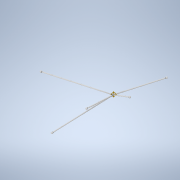
# Autodesk Inventor part: Coupler
Saved by Autodesk Inventor 2020.1 (Build 241239000, 239)
## iProperties
Created: 2019-10-25
Part Number: Coupler
Material: Generic
Document SubType Name: Modeling
Designer: sshel
Density: 1 g/cm^3
Appearance: Default
Mass: 190025 g
Surface Area: 74701 cm^2
Volume: 190025 cm^3
Author: sshel
Autodesk Inventor part; units mm, degrees
ref_plane "YZ Plane" through (0, 0, 0) normal (1, 0, 0) x (0, 1, 0)
ref_plane "XZ Plane" through (0, 0, 0) normal (0, 1, 0) x (-1, 0, 0)
ref_plane "XY Plane" through (0, 0, 0) normal (0, 0, 1) x (1, 0, 0)
ref_plane "Dyad1 plane" through (-2903, -72.8, 218.4) normal (-0.9968703, -0.024999, 0.0749971) x (0.0250696, -0.9996857, 0)
sketch "Sketch3" plane through (-2903, -72.8, 218.4) normal (-0.9968703, -0.024999, 0.0749971) x (0.0250696, -0.9996857, 0)
  circle A0 centre (0, 0) radius 50
  point P0 (0, 0)
  dimension "d16" = 50
  constraints: 1 centre point, 1 coincident
  measures "d16" radius of A0
sketch3d "import_point_3Dsketch"
  line L0 (-2903, -72.8, 218.4) -> (0, 0, 0)
sweep "Dyad1 rod" add profiles "Sketch3" path "import_point_3Dsketch"
sketch "Sketch2" plane through (-2903, -72.8, 218.4) normal (-0.9968703, -0.024999, 0.0749971) x (0.0250696, -0.9996857, 0)
  circle A0 centre (0, 0) radius 100
  line L0 (100, 0) -> (-100, 0)
  point P0 (0, 0)
  dimension "d17" = 100
  constraints: 2 end point, 2 point on circle, 1 centre point, 1 coincident, 1 horizontal, 1 midpoint
  measures "d17" radius of A0
revolve "Dyad1 joint" add sketch "Sketch2" angle 360 about axis through (-2900.493, -172.7686, 218.4) along (-0.0250696, 0.9996857, 0) separate body picked at (-20.1483, -40.7644) contours A0 L0
ref_plane "Dyad2 plane" through (-331.6, -2095.8, 1005.2) normal (-0.1412309, -0.892617, 0.4281223) x (0.9877132, -0.1562772, 0)
sketch "Sketch4" plane through (-331.6, -2095.8, 1005.2) normal (-0.1412309, -0.892617, 0.4281223) x (0.9877132, -0.1562772, 0)
  circle A0 centre (0, 0) radius 50
  dimension "d14" = 50
  constraints: 1 centre point, 1 coincident
  measures "d14" radius of A0
sketch3d "import_point_3Dsketch for Dyad2 rod"
  line L0 (-331.6, -2095.8, 1005.2) -> (0, 0, 0)
sweep "Dyad2 rod" add profiles "Sketch4" path "import_point_3Dsketch for Dyad2 rod" separate body
sketch "Sketch5" plane through (-331.6, -2095.8, 1005.2) normal (-0.1412309, -0.892617, 0.4281223) x (0.9877132, -0.1562772, 0)
  circle A0 centre (0, 0) radius 100
  line L0 (100, 0) -> (-100, 0)
  dimension "d11" = 100
  constraints: 2 end point, 2 point on circle, 1 centre point, 1 coincident, 1 horizontal, 1 midpoint
  measures "d11" radius of A0
revolve "Dyad2 joint" add sketch "Sketch5" angle 360 about axis through (-232.8287, -2111.4277, 1005.2) along (-0.9877132, 0.1562772, 0) picked at (-20.1483, -40.7644) bodies 2 contours A0 L0
ref_plane "Dyad3 plane" through (-5519.4, 1007.5, -1258) normal (-0.9599117, 0.1752203, -0.2187863) x (-0.1795708, -0.9837451, 0)
sketch "Sketch6" plane through (-5519.4, 1007.5, -1258) normal (-0.9599117, 0.1752203, -0.2187863) x (-0.1795708, -0.9837451, 0)
  circle A0 centre (0, 0) radius 50
  point P0 (0, 0)
  dimension "d18" = 50
  constraints: 1 centre point, 1 coincident
  measures "d18" radius of A0
sketch3d "import_point_3Dsketch for Dyad3 rod"
  line L0 (-5519.4, 1007.5, -1258) -> (0, 0, 0)
sweep "Dyad3 rod" add profiles "Sketch6" path "import_point_3Dsketch for Dyad3 rod" separate body
sketch "Sketch7" plane through (-5519.4, 1007.5, -1258) normal (-0.9599117, 0.1752203, -0.2187863) x (-0.1795708, -0.9837451, 0)
  circle A0 centre (0, 0) radius 100
  line L0 (100, 0) -> (-100, 0)
  point P0 (0, 0)
  dimension "d21" = 100
  constraints: 2 end point, 2 point on circle, 1 centre point, 1 coincident, 1 horizontal, 1 midpoint
  measures "d21" radius of A0
revolve "Dyad3 joint" add sketch "Sketch7" angle 360 about axis through (-5537.3571, 909.1255, -1258) along (0.1795708, 0.9837451, 0) picked at (-20.1483, -40.7644) bodies 2 contours A0 L0
ref_plane "Dyad4 plane" through (4188.4, -1511.9, 245.4) normal (0.9391702, -0.3390153, 0.0550264) x (0.3395297, 0.9405953, 0)
sketch "Sketch8" plane through (4188.4, -1511.9, 245.4) normal (0.9391702, -0.3390153, 0.0550264) x (0.3395297, 0.9405953, 0)
  circle A0 centre (0, 0) radius 50
  point P0 (0, 0)
  dimension "d23" = 50
  constraints: 1 centre point, 1 coincident
  measures "d23" radius of A0
sketch3d "import_point_3Dsketch for Dyad4 rod"
  line L0 (4188.4, -1511.9, 245.4) -> (0, 0, 0)
sweep "Dyad4 rod" add profiles "Sketch8" path "import_point_3Dsketch for Dyad4 rod" separate body
sketch "Sketch9" plane through (4188.4, -1511.9, 245.4) normal (0.9391702, -0.3390153, 0.0550264) x (0.3395297, 0.9405953, 0)
  circle A0 centre (0, 0) radius 100
  line L0 (100, 0) -> (-100, 0)
  point P0 (0, 0)
  dimension "d26" = 100
  constraints: 2 end point, 2 point on circle, 1 centre point, 1 coincident, 1 horizontal, 1 midpoint
  measures "d26" radius of A0
revolve "Dyad4 joint" add sketch "Sketch9" angle 360 about axis through (4222.353, -1417.8405, 245.4) along (-0.3395297, -0.9405953, 0) picked at (-20.1483, -40.7644) bodies 2 contours A0 L0
ref_plane "Dyad5 plane" through (-1998.5, 5711.8, 293.6) normal (-0.3298696, 0.9427818, 0.0484612) x (-0.9438908, -0.3302577, 0)
sketch "Sketch10" plane through (-1998.5, 5711.8, 293.6) normal (-0.3298696, 0.9427818, 0.0484612) x (-0.9438908, -0.3302577, 0)
  circle A0 centre (0, 0) radius 50
  point P0 (0, 0)
  dimension "d28" = 50
  constraints: 1 centre point, 1 coincident
  measures "d28" radius of A0
sketch3d "import_point_3Dsketch for Dyad5 rod"
  line L0 (-1998.5, 5711.8, 293.6) -> (0, 0, 0)
sweep "Dyad5 rod" add profiles "Sketch10" path "import_point_3Dsketch for Dyad5 rod" separate body
sketch "Sketch11" plane through (-1998.5, 5711.8, 293.6) normal (-0.3298696, 0.9427818, 0.0484612) x (-0.9438908, -0.3302577, 0)
  circle A0 centre (0, 0) radius 100
  line L0 (100, 0) -> (-100, 0)
  point P0 (0, 0)
  dimension "d31" = 100
  constraints: 2 end point, 2 point on circle, 1 centre point, 1 coincident, 1 horizontal, 1 midpoint
  measures "d31" radius of A0
revolve "Dyad5 joint" add sketch "Sketch11" angle 360 about axis through (-2092.8891, 5678.7742, 293.6) along (0.9438908, 0.3302577, 0) picked at (-20.1483, -40.7644) bodies 2 contours A0 L0
combine bodies "Combine1" operation type add bodies to combine 1 2 3 4 5 6
sketch "Sketch12" plane through (0, 0, 0) normal (0, 0, 1) x (1, 0, 0)
  circle A0 centre (0, 0) radius 100
  line L0 (-100, 0) -> (100, 0)
  dimension "d33" = 200
  constraints: 2 end point, 2 point on circle, 1 centre point, 1 coincident, 1 horizontal, 1 midpoint
  measures "d33" diameter of A0
revolve "Revolution7" add sketch "Sketch12" angle 360 about axis through (-100, 0, 0) along (1, 0, 0) picked at (-20.1483, -40.7644) bodies 1 contours A0 L0
equation "\"d16\" = rod_radius"
equation "\"d17\" = S_radius"
equation "\"d14\" = rod_radius"
equation "\"d11\" = S_radius"
equation "\"d18\" = rod_radius"
equation "\"d21\" = S_radius"
equation "\"d23\" = rod_radius"
equation "\"d26\" = S_radius"
equation "\"d28\" = rod_radius"
equation "\"d31\" = S_radius"
equation "\"d33\" = 2 * S_radius"
equation "\"rod_radius\" = 50"
equation "\"S_radius\" = 2 * rod_radius"
body "Solid3"
